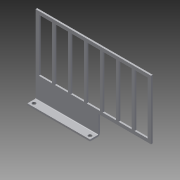
# Autodesk Inventor part: Wall
Saved by Autodesk Inventor 2013 (Build 170138000, 138)
## iProperties
Created: 2013-02-01
Part Number: Wall
Material: Aluminum 6061
Document SubType Name: Sheet Metal
Designer: actoennies
Mass: 272.717 g
Surface Area: 659.98 cm^2
Volume: 100.633 cm^3
Density: 2.71 g/cm^3
Sheet Metal Rule: Default
Flat Pattern Width: 11.5949 cm
Flat Pattern Length: 22.225 cm
Flat Pattern Area: 257.697 cm^2
Sheet Metal Width: 4.565 in
Sheet Metal Length: 8.750 in
Sheet Metal Area: 39.943 in^2
Author: actoennies
Autodesk Inventor part; units mm, degrees
ref_plane "YZ Plane" through (0, 0, 0) normal (1, 0, 0) x (0, 1, 0)
ref_plane "XZ Plane" through (0, 0, 0) normal (0, 1, 0) x (-1, 0, 0)
ref_plane "XY Plane" through (0, 0, 0) normal (0, 0, 1) x (1, 0, 0)
sketch "Sketch1" plane through (0, 0, 0) normal (0, 1, 0) x (-1, 0, 0)
  line L0 (0, 0) -> (0, 19.05)
  line L1 (0, 19.05) -> (120.65, 19.05)
  line L2 (120.65, 19.05) -> (120.65, 0)
  line L3 (120.65, 0) -> (0, 0)
  circle A0 centre (6.35, 12.7) radius 3.3782
  circle A1 centre (114.3, 12.7) radius 3.3782
  dimension "d0" = 19.05
  dimension "d1" = 120.65
  dimension "d2" = 6.7564
  dimension "d3" = 6.7564
  dimension "d4" = 107.95
  dimension "d5" = 6.35
  dimension "d6" = 12.7
  dimension "d7" = 12.7
extrude "Plate1" add sketch "Sketch1" along normal blind 3.175
sketch "Sketch2" plane through (-120.65, 0, 3.175) normal (0, 0, -1) x (-1, 0, 0)
  line L0 (-120.65, 0) -> (0, 0)
  line L1 (0, 0) -> (0, 38.1)
  line L2 (0, 38.1) -> (-120.65, 38.1)
  line L3 (-120.65, 38.1) -> (-120.65, 0)
  constraints: 6 end point, 1 horizontal, 1 perpendicular, 1 vertical
edge flange "Flange1" height 38.1 angle 90 thickness 3.175 bend radius 1.27 thickness toward (0, 0, -1) relief straight relief width 3.175 relief depth 1.5875 edges at (-60.325, 3.175, 0) wall of the first edge with corners at (0, 0, 3.175) (-120.65, 0, 3.175) (-120.65, 38.1, 3.175) (0, 38.1, 3.175)
bend "Bend1"
corner "Corner1"
sketch "Sketch3" plane through (-120.65, 38.1, 3.175) normal (0, 0, 1) x (1, 0, 0)
  line L0 (120.65, 0) -> (0, 0) projected
  line L1 (120.65, 0) -> (120.65, -33.655) projected
  line L2 (0, 0) -> (0, 63.5)
  line L3 (0, 63.5) -> (120.65, 63.5)
  line L4 (120.65, 63.5) -> (222.25, 63.5)
  line L5 (222.25, 63.5) -> (222.25, 0)
  line L6 (222.25, 0) -> (120.65, 0)
  point P0 (120.65, -38.1)
  dimension "d42" = 63.5
  dimension "d43" = 101.6
  constraints: 10 end point, 3 parallel, 1 collinear, 1 perpendicular
  measures "d42" distance of L0.end L2.end
  measures "d43" distance of L3.end L4.end
sheet face with bend "Face2" sketch "Sketch3" thickness 3.175 toward (0, 0, -1) bend radius 3.175 relief straight relief width 3.175 relief depth 1.5875
bend "Bend2"
sketch "Sketch5" plane through (-120.65, 4.445, 3.175) normal (0, 0, 1) x (1, 0, 0)
  line L0 (222.25, 33.655) -> (120.65, 33.655) projected
  line L1 (222.25, 97.155) -> (222.25, 33.655) projected
  line L2 (0, 97.155) -> (222.25, 97.155) projected
  line L3 (215.9, 90.805) -> (215.9, 40.005)
  line L4 (215.9, 40.005) -> (190.5, 40.005)
  line L5 (190.5, 40.005) -> (190.5, 90.805)
  line L6 (190.5, 90.805) -> (215.9, 90.805)
  line L7 (185.2083, 90.805) -> (185.2083, 40.005)
  line L8 (185.2083, 40.005) -> (159.8083, 40.005)
  line L9 (159.8083, 40.005) -> (159.8083, 90.805)
  line L10 (159.8083, 90.805) -> (185.2083, 90.805)
  line L11 (154.5167, 90.805) -> (154.5167, 40.005)
  line L12 (154.5167, 40.005) -> (129.1167, 40.005)
  line L13 (129.1167, 40.005) -> (129.1167, 90.805)
  line L14 (129.1167, 90.805) -> (154.5167, 90.805)
  line L15 (123.825, 90.805) -> (123.825, 40.005)
  line L16 (123.825, 40.005) -> (98.425, 40.005)
  line L17 (98.425, 40.005) -> (98.425, 90.805)
  line L18 (98.425, 90.805) -> (123.825, 90.805)
  line L19 (93.1333, 90.805) -> (93.1333, 40.005)
  line L20 (93.1333, 40.005) -> (67.7333, 40.005)
  line L21 (67.7333, 40.005) -> (67.7333, 90.805)
  line L22 (67.7333, 90.805) -> (93.1333, 90.805)
  line L23 (62.4417, 90.805) -> (62.4417, 40.005)
  line L24 (62.4417, 40.005) -> (37.0417, 40.005)
  line L25 (37.0417, 40.005) -> (37.0417, 90.805)
  line L26 (37.0417, 90.805) -> (62.4417, 90.805)
  line L27 (31.75, 90.805) -> (31.75, 40.005)
  line L28 (31.75, 40.005) -> (6.35, 40.005)
  line L29 (6.35, 40.005) -> (6.35, 90.805)
  line L30 (6.35, 90.805) -> (31.75, 90.805)
  point P0 (120.65, -4.445)
  dimension "d44" = 50.8
  dimension "d45" = 25.4
  dimension "d46" = 6.35
  dimension "d47" = 6.35
  dimension "d50" = 30.6917
  constraints: 56 end point, 2 parallel, 2 perpendicular, 1 horizontal, 48 other
  measures "d44" distance of L3.start L3.end
  measures "d45" distance of L3.end L4.end
  measures "d46" distance from line of L2 L3.start
  measures "d47" distance from line of L1 L3.start
  measures "d50" distance of L3.start L7.start
extrude "Cut2" cut sketch "Sketch5" against normal blind 3.175
equation "\"d55\" = Thickness"
equation "\"d9\" = BendReliefWidth"
equation "\"d10\" = BendReliefDepth"
equation "\"d11\" = MinimumRemnant"
equation "\"d12\" = BendRadius"
equation "\"d16\" = CornerReliefSize"
equation "\"d17\" = GapSize"
equation "\"d18\" = JacobiRadiusSize"
equation "\"d21\" = BendRadius"
equation "\"d22\" = BendReliefWidth"
equation "\"d24\" = MinimumRemnant"
equation "\"d23\" = BendReliefDepth"
equation "\"d25\" = BendRadius"
equation "\"BendRadius\" = Thickness"
equation "\"BendReliefWidth\" = Thickness"
equation "\"BendReliefDepth\" = 0.5 * Thickness"
equation "\"CornerReliefSize\" = 4 * Thickness"
equation "\"MinimumRemnant\" = 2 * Thickness"
equation "\"TransitionRadius\" = BendRadius"
equation "\"JacobiRadiusSize\" = BendRadius"
equation "\"GapSize\" = Thickness"
equation "\"d8\" = BendRadius"
equation "\"Thickness\" = 3.175"
body "Solid1"
